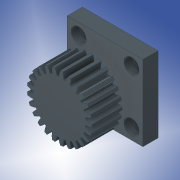
# Autodesk Inventor part: BA007
Saved by Autodesk Inventor 2017 (Build 210142000, 142)
## iProperties
Created: 2017-06-15
Part Number: BA007
Material: ABS Plastic
Document SubType Name: Modeling
Designer: zallen
Density: 1.06 g/cm^3
Appearance: CR Dark Blue
Author: zallen
Autodesk Inventor part; units mm, degrees
ref_plane "YZ Plane" through (0, 0, 0) normal (1, 0, 0) x (0, 1, 0)
ref_plane "XZ Plane" through (0, 0, 0) normal (0, 1, 0) x (-1, 0, 0)
ref_plane "XY Plane" through (0, 0, 0) normal (0, 0, 1) x (1, 0, 0)
sketch "Sketch1" plane through (0, 0, 0) normal (0, 0, 1) x (1, 0, 0)
  line L0 (0, 0) -> (50, 0)
  line L1 (50, 0) -> (50, 50)
  line L2 (50, 50) -> (0, 50)
  line L3 (0, 50) -> (0, 0)
  dimension "d0" = 50
  dimension "d1" = 50
  constraints: 8 end point, 2 parallel, 1 horizontal, 1 perpendicular
  measures "d0" distance of L2.end L1.end
  measures "d1" distance of L1.end L0.end
extrude "Extrusion1" add sketch "Sketch1" along normal blind 10
sketch "Sketch2" plane through (0, 0, 10) normal (0, 0, 1) x (1, 0, 0)
  line L0 (0, 50) -> (0, 0) construction
  line L1 (0, 25) -> (50, 25) construction
  line L2 (50, 0) -> (50, 50) construction
  line L3 (50, 50) -> (0, 50) construction
  line L4 (25, 50) -> (25, 0) construction
  line L5 (0, 0) -> (50, 0) construction
  line L6 (7.5, 7.5) -> (42.5, 7.5) construction
  line L7 (42.5, 7.5) -> (42.5, 42.5) construction
  line L8 (42.5, 42.5) -> (7.5, 42.5) construction
  line L9 (7.5, 42.5) -> (7.5, 7.5) construction
  line L10 (7.5, 7.5) -> (42.5, 42.5) construction
  line L11 (42.5, 7.5) -> (7.5, 42.5) construction
  circle A0 centre (42.5, 42.5) radius 2.5
  circle A1 centre (42.5, 7.5) radius 2.5
  circle A2 centre (7.5, 7.5) radius 2.5
  circle A3 centre (7.5, 42.5) radius 2.5
  point P0 (25, 25)
  dimension "d4" = 35
  dimension "d5" = 35
  dimension "d6" = 5
  dimension "d7" = 5
  dimension "d8" = 5
  dimension "d9" = 5
  constraints: 16 end point, 8 midpoint, 4 centre point, 4 coincident, 2 horizontal, 2 parallel, 1 perpendicular, 1 vertical
  measures "d4" distance of L8.end L7.end
  measures "d5" distance of L7.end L6.end
  measures "d6" diameter of A0
  measures "d7" diameter of A1
  measures "d8" diameter of A2
  measures "d9" diameter of A3
extrude "Extrusion2" cut sketch "Sketch2" against normal through all
sketch "Sketch3" plane through (0, 0, 10) normal (0, 0, 1) x (1, 0, 0)
  circle A0 centre (25, 25) radius 5
  line L0 (0, 50) -> (0, 0) projected
  line L1 (50, 50) -> (0, 50) projected
  point P0 (0, 25)
  point P1 (25, 50)
  dimension "d12" = 10
  constraints: 2 midpoint, 1 centre point, 1 horizontal alignment, 1 vertical alignment
  measures "d12" diameter of A0
extrude "Extrusion3" add sketch "Sketch3" along normal blind 10
sketch "Sketch4" plane through (25, 25, 20) normal (0, 0, 1) x (1, 0, 0)
  circle A0 centre (-0.1176, 0.006) radius 17.5
  arc A1 (21.3023, 0.906) -> (17.3023, 1.679) centre (16.4827, -13.2986) ccw
  arc A2 (17.3023, -1.6669) -> (21.3023, -0.894) centre (16.4827, 13.3107) ccw
  arc A3 (21.3023, -0.894) -> (21.3023, 0.906) centre (1.3225, 0.006) ccw
  line L0 (-0.1176, 0.006) -> (29.0806, 0.006) construction
  arc A4 (17.3023, -1.6669) -> (17.3023, 1.679) centre (-0.1176, 0.006) ccw
  arc A5 (20.4055, 6.2046) -> (16.3389, 5.9585) centre (19.2699, -8.7523) ccw
  arc A6 (20.8531, 4.4612) -> (20.4055, 6.2046) centre (1.2773, 0.3641) ccw
  arc A7 (17.171, 2.7178) -> (20.8531, 4.4612) centre (12.6524, 17.021) ccw
  circle A8 centre (-0.1176, 0.006) radius 17.5
  arc A9 (17.171, 2.7178) -> (16.3389, 5.9585) centre (-0.1176, 0.006) ccw
  arc A10 (18.2192, 11.1138) -> (14.3416, 9.8641) centre (20.8389, -3.6557) ccw
  arc A11 (19.0863, 9.5364) -> (18.2192, 11.1138) centre (1.1444, 0.6998) ccw
  arc A12 (15.9535, 6.9321) -> (19.0863, 9.5364) centre (8.0198, 19.6622) ccw
  circle A13 centre (-0.1176, 0.006) radius 17.5
  arc A14 (15.9535, 6.9321) -> (14.3416, 9.8641) centre (-0.1176, 0.006) ccw
  arc A15 (14.8807, 15.325) -> (11.4357, 13.1502) centre (21.0912, 1.671) ccw
  arc A16 (16.1129, 14.0128) -> (14.8807, 15.325) centre (0.9322, 0.9918) ccw
  arc A17 (13.7261, 10.7112) -> (16.1129, 14.0128) centre (2.8758, 21.0684) ccw
  circle A18 centre (-0.1176, 0.006) radius 17.5
  arc A19 (13.7261, 10.7112) -> (11.4357, 13.1502) centre (-0.1176, 0.006) ccw
  arc A20 (10.5998, 18.5736) -> (7.8039, 15.6105) centre (20.0108, 6.8931) ccw
  arc A21 (12.1196, 17.6091) -> (10.5998, 18.5736) centre (0.6541, 1.2219) ccw
  arc A22 (10.6289, 13.8177) -> (12.1196, 17.6091) centre (-2.4562, 21.1511) ccw
  circle A23 centre (-0.1176, 0.006) radius 17.5
  arc A24 (10.6289, 13.8177) -> (7.8039, 15.6105) centre (-0.1176, 0.006) ccw
  arc A25 (5.6456, 20.6556) -> (3.6744, 17.0902) centre (17.6656, 11.6825) ccw
  arc A26 (7.3575, 20.0994) -> (5.6456, 20.6556) centre (0.3274, 1.3756) ccw
  arc A27 (6.8565, 16.0563) -> (7.3575, 20.0994) centre (-7.6413, 19.9052) ccw
  circle A28 centre (-0.1176, 0.006) radius 17.5
  arc A29 (6.8565, 16.0563) -> (3.6744, 17.0902) centre (-0.1176, 0.006) ccw
  arc A30 (0.3291, 21.4401) -> (-0.6934, 17.4965) centre (14.2031, 15.7381) ccw
  arc A31 (2.1256, 21.3271) -> (0.3291, 21.4401) centre (-0.0272, 1.4433) ccw
  arc A32 (2.6459, 17.2864) -> (2.1256, 21.3271) centre (-12.3536, 17.409) ccw
  circle A33 centre (-0.1176, 0.006) radius 17.5
  arc A34 (2.6459, 17.2864) -> (-0.6934, 17.4965) centre (-0.1176, 0.006) ccw
  arc A35 (-5.0153, 20.8778) -> (-5.0251, 16.8038) centre (9.8408, 18.8053) ccw
  arc A36 (-3.2472, 21.2151) -> (-5.0153, 20.8778) centre (-0.3874, 1.4206) ccw
  arc A37 (-1.7384, 17.4308) -> (-3.2472, 21.2151) centre (-16.2972, 13.8192) ccw
  circle A38 centre (-0.1176, 0.006) radius 17.5
  arc A39 (-1.7384, 17.4308) -> (-5.0251, 16.8038) centre (-0.1176, 0.006) ccw
  arc A40 (-10.0521, 19.0041) -> (-9.0483, 15.0557) centre (4.8527, 20.6913) ccw
  arc A41 (-8.4234, 19.7705) -> (-10.0521, 19.0041) centre (-0.7308, 1.3091) ccw
  arc A42 (-6.0209, 16.4803) -> (-8.4234, 19.7705) centre (-19.2241, 9.3616) ccw
  circle A43 centre (-0.1176, 0.006) radius 17.5
  arc A44 (-6.0209, 16.4803) -> (-9.0483, 15.0557) centre (-0.1176, 0.006) ccw
  arc A45 (-14.4646, 15.9366) -> (-12.5105, 12.3619) centre (-0.4476, 21.2775) ccw
  arc A46 (-13.0777, 17.084) -> (-14.4646, 15.9366) centre (-1.0356, 1.1156) ccw
  arc A47 (-9.9324, 14.4946) -> (-13.0777, 17.084) centre (-20.9504, 4.3161) ccw
  circle A48 centre (-0.1176, 0.006) radius 17.5
  arc A49 (-9.9324, 14.4946) -> (-12.5105, 12.3619) centre (-0.1176, 0.006) ccw
  arc A50 (-17.9756, 11.8682) -> (-15.1939, 8.8917) centre (-5.7273, 20.5271) ccw
  arc A51 (-16.9176, 13.3244) -> (-17.9756, 11.8682) centre (-1.2827, 0.8525) ccw
  arc A52 (-13.2272, 11.5986) -> (-16.9176, 13.3244) centre (-21.3678, -1.0003) ccw
  circle A53 centre (-0.1176, 0.006) radius 17.5
  arc A54 (-13.2272, 11.5986) -> (-15.1939, 8.8917) centre (-0.1176, 0.006) ccw
  arc A55 (-20.3646, 7.0544) -> (-16.93, 4.8632) centre (-10.6544, 18.4873) ccw
  arc A56 (-19.702, 8.728) -> (-20.3646, 7.0544) centre (-1.4566, 0.5361) ccw
  arc A57 (-15.6983, 7.9742) -> (-19.702, 8.728) centre (-20.4499, -6.2534) ccw
  circle A58 centre (-0.1176, 0.006) radius 17.5
  arc A59 (-15.6983, 7.9742) -> (-16.93, 4.8632) centre (-0.1176, 0.006) ccw
  arc A60 (-21.4813, 1.7977) -> (-17.6098, 0.5295) centre (-14.9195, 15.2863) ccw
  arc A61 (-21.2557, 3.5835) -> (-21.4813, 1.7977) centre (-1.5464, 0.1865) ccw
  arc A62 (-17.1904, 3.849) -> (-21.2557, 3.5835) centre (-18.2545, -11.1132) ccw
  circle A63 centre (-0.1176, 0.006) radius 17.5
  arc A64 (-17.1904, 3.849) -> (-17.6098, 0.5295) centre (-0.1176, 0.006) ccw
  arc A65 (-21.2557, -3.5715) -> (-17.1904, -3.837) centre (-18.2545, 11.1252) ccw
  arc A66 (-21.4813, -1.7857) -> (-21.2557, -3.5715) centre (-1.5464, -0.1745) ccw
  arc A67 (-17.6098, -0.5175) -> (-21.4813, -1.7857) centre (-14.9195, -15.2743) ccw
  circle A68 centre (-0.1176, 0.006) radius 17.5
  arc A69 (-17.6098, -0.5175) -> (-17.1904, -3.837) centre (-0.1176, 0.006) ccw
  arc A70 (-19.702, -8.716) -> (-15.6983, -7.9621) centre (-20.4499, 6.2654) ccw
  arc A71 (-20.3646, -7.0424) -> (-19.702, -8.716) centre (-1.4566, -0.5241) ccw
  arc A72 (-16.93, -4.8512) -> (-20.3646, -7.0424) centre (-10.6544, -18.4753) ccw
  circle A73 centre (-0.1176, 0.006) radius 17.5
  arc A74 (-16.93, -4.8512) -> (-15.6983, -7.9621) centre (-0.1176, 0.006) ccw
  arc A75 (-16.9176, -13.3124) -> (-13.2272, -11.5866) centre (-21.3678, 1.0123) ccw
  arc A76 (-17.9756, -11.8562) -> (-16.9176, -13.3124) centre (-1.2827, -0.8405) ccw
  arc A77 (-15.1939, -8.8797) -> (-17.9756, -11.8562) centre (-5.7273, -20.5151) ccw
  circle A78 centre (-0.1176, 0.006) radius 17.5
  arc A79 (-15.1939, -8.8797) -> (-13.2272, -11.5866) centre (-0.1176, 0.006) ccw
  arc A80 (-13.0777, -17.072) -> (-9.9324, -14.4826) centre (-20.9504, -4.304) ccw
  arc A81 (-14.4646, -15.9246) -> (-13.0777, -17.072) centre (-1.0356, -1.1036) ccw
  arc A82 (-12.5105, -12.3498) -> (-14.4646, -15.9246) centre (-0.4476, -21.2654) ccw
  circle A83 centre (-0.1176, 0.006) radius 17.5
  arc A84 (-12.5105, -12.3498) -> (-9.9324, -14.4826) centre (-0.1176, 0.006) ccw
  arc A85 (-8.4234, -19.7585) -> (-6.0209, -16.4683) centre (-19.2241, -9.3496) ccw
  arc A86 (-10.0521, -18.9921) -> (-8.4234, -19.7585) centre (-0.7308, -1.297) ccw
  arc A87 (-9.0483, -15.0436) -> (-10.0521, -18.9921) centre (4.8527, -20.6792) ccw
  circle A88 centre (-0.1176, 0.006) radius 17.5
  arc A89 (-9.0483, -15.0436) -> (-6.0209, -16.4683) centre (-0.1176, 0.006) ccw
  arc A90 (-3.2472, -21.2031) -> (-1.7384, -17.4188) centre (-16.2972, -13.8072) ccw
  arc A91 (-5.0153, -20.8658) -> (-3.2472, -21.2031) centre (-0.3874, -1.4086) ccw
  arc A92 (-5.0251, -16.7918) -> (-5.0153, -20.8658) centre (9.8408, -18.7933) ccw
  circle A93 centre (-0.1176, 0.006) radius 17.5
  arc A94 (-5.0251, -16.7918) -> (-1.7384, -17.4188) centre (-0.1176, 0.006) ccw
  arc A95 (2.1256, -21.3151) -> (2.6459, -17.2744) centre (-12.3536, -17.3969) ccw
  arc A96 (0.3291, -21.4281) -> (2.1256, -21.3151) centre (-0.0272, -1.4313) ccw
  arc A97 (-0.6934, -17.4845) -> (0.3291, -21.4281) centre (14.2031, -15.7261) ccw
  circle A98 centre (-0.1176, 0.006) radius 17.5
  arc A99 (-0.6934, -17.4845) -> (2.6459, -17.2744) centre (-0.1176, 0.006) ccw
  arc A100 (7.3575, -20.0874) -> (6.8565, -16.0443) centre (-7.6413, -19.8932) ccw
  arc A101 (5.6456, -20.6436) -> (7.3575, -20.0874) centre (0.3274, -1.3636) ccw
  arc A102 (3.6744, -17.0782) -> (5.6456, -20.6436) centre (17.6656, -11.6705) ccw
  circle A103 centre (-0.1176, 0.006) radius 17.5
  arc A104 (3.6744, -17.0782) -> (6.8565, -16.0443) centre (-0.1176, 0.006) ccw
  arc A105 (12.1196, -17.5971) -> (10.6289, -13.8057) centre (-2.4562, -21.1391) ccw
  arc A106 (10.5998, -18.5616) -> (12.1196, -17.5971) centre (0.6541, -1.2099) ccw
  arc A107 (7.8039, -15.5985) -> (10.5998, -18.5616) centre (20.0108, -6.8811) ccw
  circle A108 centre (-0.1176, 0.006) radius 17.5
  arc A109 (7.8039, -15.5985) -> (10.6289, -13.8057) centre (-0.1176, 0.006) ccw
  arc A110 (16.1129, -14.0008) -> (13.7261, -10.6992) centre (2.8758, -21.0564) ccw
  arc A111 (14.8807, -15.313) -> (16.1129, -14.0008) centre (0.9322, -0.9798) ccw
  arc A112 (11.4357, -13.1382) -> (14.8807, -15.313) centre (21.0912, -1.659) ccw
  circle A113 centre (-0.1176, 0.006) radius 17.5
  arc A114 (11.4357, -13.1382) -> (13.7261, -10.6992) centre (-0.1176, 0.006) ccw
  arc A115 (19.0863, -9.5244) -> (15.9535, -6.9201) centre (8.0198, -19.6502) ccw
  arc A116 (18.2192, -11.1018) -> (19.0863, -9.5244) centre (1.1444, -0.6878) ccw
  arc A117 (14.3416, -9.8521) -> (18.2192, -11.1018) centre (20.8389, 3.6677) ccw
  circle A118 centre (-0.1176, 0.006) radius 17.5
  arc A119 (14.3416, -9.8521) -> (15.9535, -6.9201) centre (-0.1176, 0.006) ccw
  arc A120 (20.8531, -4.4492) -> (17.171, -2.7057) centre (12.6524, -17.009) ccw
  arc A121 (20.4055, -6.1926) -> (20.8531, -4.4492) centre (1.2773, -0.3521) ccw
  arc A122 (16.3389, -5.9465) -> (20.4055, -6.1926) centre (19.2699, 8.7643) ccw
  circle A123 centre (-0.1176, 0.006) radius 17.5
  arc A124 (16.3389, -5.9465) -> (17.171, -2.7057) centre (-0.1176, 0.006) ccw
  point P0 (-25, -25)
  dimension "d15" = 35
  dimension "d17" = 15
  dimension "d18" = 4
  dimension "d19" = 15
  dimension "d20" = 20
  dimension "d21" = 1.8
  dimension "d24" = 360
  constraints: 250 point on circle, 125 centre point, 2 coincident, 2 end point, 2 symmetric about line, 1 concentric, 1 horizontal, 349 other
  measures "d15" diameter of A0
  measures "d17" radius of A1
  measures "d18" horizontal distance of A1.start A0.start
  measures "d19" radius of A2
  measures "d20" radius of A3
  measures "d21" distance of A2.end A1.start
extrude "Extrusion4" add sketch "Sketch4" along normal blind 20
sketch "Sketch5" plane through (0, 0, 10) normal (0, 0, 1) x (1, 0, 0)
  circle A0 centre (25, 25) radius 5 projected
  circle A1 centre (7.5, 7.5) radius 2.5 projected
  circle A2 centre (42.5, 42.5) radius 2.5 projected
  circle A3 centre (42.5, 7.5) radius 2.5 projected
  circle A4 centre (7.5, 42.5) radius 2.5 projected
  line L0 (0, 0) -> (50, 0) projected
  line L1 (50, 0) -> (50, 50) projected
  line L2 (50, 50) -> (0, 50) projected
  line L3 (0, 50) -> (0, 0) projected
  circle A5 centre (7.5, 42.5) radius 5
  circle A6 centre (42.5, 42.5) radius 5
  circle A7 centre (42.5, 7.5) radius 5
  circle A8 centre (7.5, 7.5) radius 2.5 projected
  circle A9 centre (7.5, 7.5) radius 5
  dimension "d28" = 10
  dimension "d29" = 10
  dimension "d30" = 10
  dimension "d31" = 10
  constraints: 4 centre point, 4 coincident
  measures "d28" diameter of A5
  measures "d29" diameter of A6
  measures "d30" diameter of A7
  measures "d31" diameter of A9
extrude "Extrusion5" cut sketch "Sketch5" against normal blind 5 contours A5 | A6 | A7 | A9
body "Solid1"
